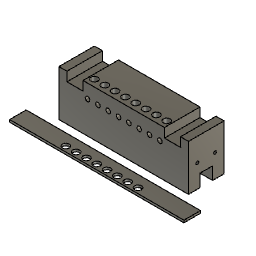
Simple_block_with_threaded_holes (Autodesk Fusion 360 design; units mm, degrees)
Autodesk Fusion 360 part; units mm, degrees
sketch "Sketch1" plane through (0, 0, 0) normal (0, 0, 1) x (1, 0, 0)
  line L0 (0, 0) -> (9, 0) construction
  line L1 (9, 0) -> (18, 0) construction
  line L2 (18, 0) -> (27, 0) construction
  line L3 (27, 0) -> (36, 0) construction
  line L4 (36, 0) -> (45, 0) construction
  line L5 (45, 0) -> (54, 0) construction
  line L6 (54, 0) -> (63, 0) construction
  line L7 (0, 0) -> (-25, 0) construction
  line L8 (63, 0) -> (88, 0) construction
  line L9 (-25, 0) -> (-25, -6) construction
  line L10 (88, 0) -> (88, -6) construction
  line L11 (88, -6) -> (-25, -6) construction
  line L12 (-25, 0) -> (-25, 25) construction
  line L13 (88, 0) -> (88, 25) construction
  line L14 (88, 25) -> (-25, 25) construction
  line L15 (88, -6) -> (-25, -6)
  line L16 (-25, -6) -> (-25, 25)
  line L17 (-25, 25) -> (88, 25)
  line L18 (88, 25) -> (88, -6)
  dimension "d1" = 9
  dimension "d2" = 9
  dimension "d3" = 9
  dimension "d4" = 9
  dimension "d5" = 9
  dimension "d6" = 9
  dimension "d7" = 9
  dimension "d8" = 25
  dimension "d9" = 25
  dimension "d10" = 6
  dimension "d11" = 6
  dimension "d12" = 25
  dimension "d13" = 25
  constraint coincident L0.start L7.start
  constraint horizontal L0
  constraint parallel L0 L1
  constraint parallel L1 L2
  constraint parallel L2 L3
  constraint parallel L3 L4
  constraint parallel L3 L5
  constraint parallel L3 L6
  constraint parallel L0 L7
  constraint parallel L6 L8
  constraint perpendicular L7 L9
  constraint perpendicular L8 L10
  constraint perpendicular L7 L12
  constraint perpendicular L8 L13
  measures "d1" distance of L0.start L0.end
  measures "d2" distance of L0.end L1.end
  measures "d3" distance of L1.end L2.end
  measures "d4" distance of L2.end L3.end
  measures "d5" distance of L3.end L4.end
  measures "d6" distance of L4.end L5.end
  measures "d7" distance of L5.end L6.end
  measures "d8" distance of L0.start L7.end
  measures "d9" distance of L6.end L8.end
  measures "d10" distance of L7.end L9.end
  measures "d11" distance of L8.end L10.end
  measures "d12" distance of L7.end L12.end
  measures "d13" distance of L8.end L13.end
  measures "d45" distance of L7.end
  measures "d53" diameter of L7.end
  measures "d91" distance of L7.end
extrude "Extrude1" add sketch "Sketch1" along normal blind 40 makes body 1
sketch "Sketch2" plane through (0, 0, 40) normal (0, 0, 1) x (-1, 0, 0)
  line L0 (-88, -25) -> (25, -25)
  line L1 (25, -25) -> (25, 6)
  line L2 (25, 6) -> (-88, 6)
  line L3 (-88, 6) -> (-88, -25)
  line L4 (25, 6) -> (25, 0) construction
  line L5 (25, 0) -> (0, 0) construction
  line L6 (0, 0) -> (-9, 0) construction
  line L7 (-9, 0) -> (-18, 0) construction
  line L8 (-18, 0) -> (-27, 0) construction
  line L9 (-27, 0) -> (-36, 0) construction
  line L10 (-36, 0) -> (-45, 0) construction
  line L11 (-45, 0) -> (-54, 0) construction
  line L12 (-54, 0) -> (-63, 0) construction
  line L13 (-63, 0) -> (-88, 0) construction
  circle A0 centre (0, 0) radius 3
  circle A1 centre (-9, 0) radius 3
  circle A2 centre (-18, 0) radius 3
  circle A3 centre (-27, 0) radius 3
  circle A4 centre (-36, 0) radius 3
  circle A5 centre (-45, 0) radius 3
  circle A6 centre (-54, 0) radius 3
  circle A7 centre (-63, 0) radius 3
  line L14 (0, 0) -> (4, 0) construction
  line L15 (0, 0) -> (18, 0) construction
  line L16 (-63, 0) -> (-81, 0) construction
  line L17 (-63, 0) -> (-67, 0) construction
  line L18 (-67, 0) -> (-67, 6) construction
  line L19 (-81, 0) -> (-81, 6) construction
  line L20 (-67, 6) -> (-67, -25)
  line L21 (-81, 6) -> (-81, -25)
  line L22 (18, 0) -> (18, 6) construction
  line L23 (4, 0) -> (4, 6) construction
  line L24 (18, 6) -> (18, -25)
  line L25 (4, 6) -> (4, -25)
  dimension "d16" = 6
  dimension "d17" = 25
  dimension "d18" = 9
  dimension "d19" = 9
  dimension "d20" = 9
  dimension "d21" = 9
  dimension "d22" = 9
  dimension "d23" = 9
  dimension "d24" = 9
  dimension "d25" = 6
  dimension "d26" = 6
  dimension "d27" = 6
  dimension "d28" = 6
  dimension "d29" = 6
  dimension "d30" = 6
  dimension "d31" = 6
  dimension "d32" = 6
  dimension "d56" = 4
  dimension "d57" = 18
  dimension "d58" = 18
  dimension "d59" = 4
  constraint coincident L1.end L2.start
  constraint perpendicular L2 L4
  constraint perpendicular L4 L5
  constraint perpendicular L4 L6
  constraint perpendicular L4 L7
  constraint parallel L7 L8
  constraint parallel L8 L9
  constraint parallel L9 L10
  constraint parallel L10 L11
  constraint parallel L11 L12
  constraint coincident L3 L13.end
  constraint perpendicular L3 L13
  constraint coincident L5.end L6.start
  constraint coincident L6.end L7.start
  constraint coincident L7.end L8.start
  constraint coincident L8.end L9.start
  constraint coincident L9.end L10.start
  constraint coincident L10.end L11.start
  constraint coincident L11.end L12.start
  constraint coincident L12.end L13.start
  constraint parallel L5 L14
  constraint parallel L5 L15
  constraint parallel L13 L16
  constraint parallel L13 L17
  constraint coincident L2 L18.end
  constraint perpendicular L2 L18
  constraint coincident L2 L19.end
  constraint perpendicular L2 L19
  constraint coincident L0 L20.end
  constraint perpendicular L0 L20
  constraint coincident L0 L21.end
  constraint perpendicular L0 L21
  constraint coincident L2 L22.end
  constraint perpendicular L2 L22
  constraint coincident L2 L23.end
  constraint perpendicular L2 L23
  constraint coincident L0 L24.end
  constraint perpendicular L0 L24
  constraint coincident L0 L25.end
  constraint perpendicular L0 L25
  measures "d16" distance of L1.end L4.end
  measures "d17" distance of L4.end L5.end
  measures "d18" distance of L5.end L6.end
  measures "d19" distance of L6.end L7.end
  measures "d20" distance of L7.end L8.end
  measures "d21" distance of L8.end L9.end
  measures "d22" distance of L9.end L10.end
  measures "d23" distance of L10.end L11.end
  measures "d24" distance of L11.end L12.end
  measures "d25" diameter of A0
  measures "d26" diameter of A1
  measures "d27" diameter of A2
  measures "d28" diameter of A3
  measures "d29" diameter of A4
  measures "d30" diameter of A5
  measures "d31" diameter of A6
  measures "d32" diameter of A7
  measures "d56" distance of L5.end L14.end
  measures "d57" distance of L5.end L15.end
  measures "d58" distance of L12.end L16.end
  measures "d59" distance of L12.end L17.end
sketch "Sketch3" plane through (0, -6, 0) normal (0, -1, 0) x (1, 0, 0)
  line L0 (-25, 0) -> (88, 0)
  line L1 (88, 0) -> (88, 40)
  line L2 (88, 40) -> (-25, 40)
  line L3 (-25, 40) -> (-25, 0)
  line L4 (-25, 40) -> (0, 40) construction
  line L5 (0, 40) -> (9, 40) construction
  line L6 (9, 40) -> (18, 40) construction
  line L7 (18, 40) -> (27, 40) construction
  line L8 (27, 40) -> (36, 40) construction
  line L9 (36, 40) -> (45, 40) construction
  line L10 (45, 40) -> (54, 40) construction
  line L11 (54, 40) -> (63, 40) construction
  line L12 (63, 40) -> (88, 40) construction
  line L13 (0, 40) -> (0, 28) construction
  line L14 (63, 40) -> (63, 28) construction
  line L15 (63, 28) -> (0, 28) construction
  line L16 (9, 40) -> (9, 28) construction
  line L17 (18, 40) -> (18, 28) construction
  line L18 (27, 40) -> (27, 28) construction
  line L19 (36, 40) -> (36, 28) construction
  line L20 (45, 40) -> (45, 28) construction
  line L21 (54, 40) -> (54, 28) construction
  circle A0 centre (0, 28) radius 2
  circle A1 centre (9, 28) radius 2
  circle A2 centre (18, 28) radius 2
  circle A3 centre (27, 28) radius 2
  circle A4 centre (36, 28) radius 2
  circle A5 centre (45, 28) radius 2
  circle A6 centre (54, 28) radius 2
  circle A7 centre (63, 28) radius 2
  dimension "d33" = 25
  dimension "d34" = 9
  dimension "d35" = 9
  dimension "d36" = 9
  dimension "d37" = 9
  dimension "d38" = 9
  dimension "d39" = 9
  dimension "d40" = 9
  dimension "d44" = 12
  dimension "d45" = 12
  dimension "d46" = 4
  dimension "d47" = 4
  dimension "d48" = 4
  dimension "d49" = 4
  dimension "d50" = 4
  dimension "d51" = 4
  dimension "d52" = 4
  dimension "d53" = 4
  constraint coincident L2.end L3.start
  constraint perpendicular L3 L4
  constraint perpendicular L3 L5
  constraint coincident L2 L6.end
  constraint parallel L2 L7
  constraint parallel L2 L8
  constraint parallel L2 L9
  constraint parallel L2 L10
  constraint parallel L2 L11
  constraint coincident L1.end L2.start
  constraint perpendicular L4 L13
  constraint perpendicular L11 L14
  constraint coincident L15 L16.end
  constraint perpendicular L15 L16
  constraint coincident L15 L17.end
  constraint perpendicular L15 L17
  constraint coincident L15 L18.end
  constraint perpendicular L15 L18
  constraint coincident L15 L19.end
  constraint perpendicular L15 L19
  constraint coincident L15 L20.end
  constraint perpendicular L15 L20
  constraint coincident L15 L21.end
  constraint perpendicular L15 L21
  constraint coincident L13.end L15.end
  constraint coincident L16.end A1.centre
  constraint coincident L17.end A2.centre
  constraint coincident L18.end A3.centre
  constraint coincident L19.end A4.centre
  constraint coincident L20.end A5.centre
  constraint coincident L21.end A6.centre
  constraint coincident L14.end L15.start
  measures "d33" distance of L2.end L4.end
  measures "d34" distance of L4.end L5.end
  measures "d35" distance of L5.end L6.end
  measures "d36" distance of L6.end L7.end
  measures "d37" distance of L7.end L8.end
  measures "d38" distance of L8.end L9.end
  measures "d39" distance of L9.end L10.end
  measures "d40" distance of L10.end L11.end
  measures "d44" distance of L4.end L13.end
  measures "d45" distance of L11.end L14.end
  measures "d46" diameter of A0
  measures "d47" diameter of A1
  measures "d48" diameter of A2
  measures "d49" diameter of A3
  measures "d50" diameter of A4
  measures "d51" diameter of A5
  measures "d52" diameter of A6
  measures "d53" diameter of A7
extrude "Extrude2" cut sketch "Sketch2" against normal blind 14 contours A0 | A1 | A2 | A3 | A4 | A5 | A6 | A7 bodies 1
extrude "Extrude3" cut sketch "Sketch3" against normal blind 6 contours A0 | A1 | A2 | A3 | A4 | A5 | A6 | A7 bodies 1
extrude "Extrude4" cut sketch "Sketch2" against normal blind 8 contours L0 L2 L20 L21 | L0 L2 L24 L25 bodies 1
sketch "Sketch4" plane through (88, 0, 0) normal (1, 0, 0) x (0, 1, 0)
  line L0 (-6, 0) -> (25, 0)
  line L1 (25, 0) -> (25, 40)
  line L2 (25, 40) -> (-6, 40)
  line L3 (-6, 40) -> (-6, 0)
  line L4 (9.5, 0) -> (9.5, 11) construction
  line L5 (9.5, 11) -> (15, 11) construction
  line L6 (15, 11) -> (9.5, 11) construction
  line L7 (9.5, 11) -> (4, 11) construction
  line L8 (4, 11) -> (4, 0)
  line L9 (15, 11) -> (15, 0)
  line L10 (15, 11) -> (4, 11)
  dimension "d62" = 11
  dimension "d63" = 5.5
  dimension "d64" = 5.5
  constraint midpoint L0 L4.start
  constraint perpendicular L0 L4
  constraint perpendicular L4 L5
  constraint perpendicular L4 L7
  constraint coincident L0 L8.end
  constraint perpendicular L0 L8
  constraint coincident L0 L9.end
  constraint perpendicular L0 L9
  measures "d62" distance of L4.start L4.end
  measures "d63" distance of L4.end L5.end
  measures "d64" distance of L4.end L7.end
extrude "Extrude5" cut sketch "Sketch4" against normal blind 113 contours L0 L8 L9 L10 bodies 1
sketch "Sketch5" plane through (88, 0, 0) normal (1, 0, 0) x (0, 1, 0)
  line L0 (15, 11) -> (15, 0)
  line L1 (15, 0) -> (25, 0)
  line L2 (25, 0) -> (25, 40)
  line L3 (25, 40) -> (-6, 40)
  line L4 (-6, 40) -> (-6, 0)
  line L5 (-6, 0) -> (4, 0)
  line L6 (4, 0) -> (4, 11)
  line L7 (4, 11) -> (15, 11)
  line L8 (-6, 40) -> (-6, 20) construction
  line L9 (-6, 20) -> (25, 20) construction
  line L10 (9.5, 20) -> (-6, 20) construction
  line L11 (9.5, 20) -> (25, 20) construction
  circle A0 centre (17.25, 20) radius 1.25
  circle A1 centre (1.75, 20) radius 1.25
  dimension "d67" = 20
  dimension "d68" = 2.5
  dimension "d69" = 2.5
  constraint coincident L3.end L4.start
  constraint midpoint L4 L8.end
  constraint midpoint L2 L9.end
  constraint midpoint L9 L10.start
  constraint midpoint L11 A0.centre
  constraint midpoint L10 A1.centre
  measures "d67" distance of L3.end L8.end
  measures "d68" diameter of A0
  measures "d69" diameter of A1
extrude "Extrude6" cut sketch "Sketch5" against normal blind 15 contours A0 | A1 bodies 1
sketch "Sketch6" plane through (-25, 0, 0) normal (-1, 0, 0) x (0, -1, 0)
  line L0 (-15, 0) -> (-15, 11)
  line L1 (-15, 11) -> (-4, 11)
  line L2 (-4, 11) -> (-4, 0)
  line L3 (-4, 0) -> (6, 0)
  line L4 (6, 0) -> (6, 40)
  line L5 (6, 40) -> (-25, 40)
  line L6 (-25, 40) -> (-25, 0)
  line L7 (-25, 0) -> (-15, 0)
  line L8 (-25, 40) -> (-25, 20) construction
  line L9 (-25, 20) -> (6, 20) construction
  line L10 (-9.5, 20) -> (6, 20) construction
  line L11 (-9.5, 20) -> (-25, 20) construction
  circle A0 centre (-17.25, 20) radius 1.25
  circle A1 centre (-1.75, 20) radius 1.25
  dimension "d72" = 20
  dimension "d73" = 2.5
  dimension "d74" = 2.5
  constraint coincident L5.end L6.start
  constraint perpendicular L5 L8
  constraint midpoint L4 L9.end
  constraint midpoint L9 L10.start
  constraint midpoint L11 A0.centre
  constraint midpoint L10 A1.centre
  measures "d72" distance of L5.end L8.end
  measures "d73" diameter of A0
  measures "d74" diameter of A1
extrude "Extrude7" cut sketch "Sketch6" against normal blind 15 contours A0 | A1 bodies 1
sketch "Sketch1 (2)" plane through (0, 0, 0) normal (0, 0, 1) x (1, 0, 0) in component "Lid"
  line L0 (0, -25) -> (9, -25) construction
  line L1 (9, -25) -> (18, -25) construction
  line L2 (18, -25) -> (27, -25) construction
  line L3 (27, -25) -> (36, -25) construction
  line L4 (36, -25) -> (45, -25) construction
  line L5 (45, -25) -> (54, -25) construction
  line L6 (54, -25) -> (63, -25) construction
  line L7 (63, -25) -> (63, -29.5) construction
  line L8 (0, -25) -> (0, -29.5) construction
  line L9 (0, -25) -> (0, -15) construction
  line L10 (63, -25) -> (63, -15) construction
  line L11 (0, -25) -> (-4.5, -25) construction
  line L12 (-4.5, -25) -> (-44.5, -25) construction
  line L13 (63, -25) -> (67.5, -25) construction
  line L14 (67.5, -25) -> (107.5, -25) construction
  line L15 (107.5, -25) -> (107.5, -29.5) construction
  line L16 (-44.5, -25) -> (-44.5, -29.5) construction
  line L17 (-44.5, -25) -> (-44.5, -15) construction
  line L18 (107.5, -25) -> (107.5, -15) construction
  line L19 (107.5, -15) -> (107.5, -29.5)
  line L20 (-44.5, -29.5) -> (-44.5, -15)
  line L21 (-44.5, -29.5) -> (107.5, -29.5)
  line L22 (107.5, -15) -> (-44.5, -15)
  circle A0 centre (0, -25) radius 3
  circle A1 centre (9, -25) radius 3
  circle A2 centre (18, -25) radius 3
  circle A3 centre (27, -25) radius 3
  circle A4 centre (36, -25) radius 3
  circle A5 centre (45, -25) radius 3
  circle A6 centre (54, -25) radius 3
  circle A7 centre (63, -25) radius 3
  dimension "d77" = 9
  dimension "d78" = 9
  dimension "d79" = 9
  dimension "d80" = 9
  dimension "d81" = 9
  dimension "d82" = 9
  dimension "d83" = 9
  dimension "d84" = 4.5
  dimension "d85" = 4.5
  dimension "d86" = 10
  dimension "d87" = 10
  dimension "d88" = 4.5
  dimension "d89" = 40
  dimension "d90" = 4.5
  dimension "d91" = 40
  dimension "d92" = 4.5
  dimension "d93" = 4.5
  dimension "d94" = 10
  dimension "d95" = 10
  dimension "d96" = 6
  dimension "d97" = 6
  dimension "d98" = 6
  dimension "d99" = 6
  dimension "d100" = 6
  dimension "d101" = 6
  dimension "d102" = 6
  dimension "d103" = 6
  constraint horizontal L0
  constraint parallel L0 L1
  constraint parallel L1 L2
  constraint parallel L2 L3
  constraint parallel L3 L4
  constraint parallel L4 L5
  constraint parallel L5 L6
  constraint perpendicular L6 L7
  constraint perpendicular L0 L8
  constraint perpendicular L0 L9
  constraint perpendicular L6 L10
  constraint perpendicular L9 L11
  constraint perpendicular L9 L12
  constraint perpendicular L7 L13
  constraint perpendicular L7 L14
  constraint perpendicular L14 L15
  constraint perpendicular L12 L16
  constraint perpendicular L12 L17
  constraint perpendicular L14 L18
  constraint coincident L0.start L8.start
  constraint coincident L0.end L1.start
  constraint coincident L1.end L2.start
  constraint coincident L2.end L3.start
  constraint coincident L3.end L4.start
  constraint coincident L4.end L5.start
  constraint coincident L5.end L6.start
  constraint coincident L6.end L7.start
  measures "d77" distance of L0.start L0.end
  measures "d78" distance of L0.end L1.end
  measures "d79" distance of L1.end L2.end
  measures "d80" distance of L2.end L3.end
  measures "d81" distance of L3.end L4.end
  measures "d82" distance of L4.end L5.end
  measures "d83" distance of L5.end L6.end
  measures "d84" distance of L6.end L7.end
  measures "d85" distance of L0.start L8.end
  measures "d86" distance of L0.start L9.end
  measures "d87" distance of L6.end L10.end
  measures "d88" distance of L0.start L11.end
  measures "d89" distance of L11.end L12.end
  measures "d90" distance of L6.end L13.end
  measures "d91" distance of L13.end L14.end
  measures "d92" distance of L14.end L15.end
  measures "d93" distance of L12.end L16.end
  measures "d94" distance of L12.end L17.end
  measures "d95" distance of L14.end L18.end
  measures "d96" diameter of A0
  measures "d97" diameter of A1
  measures "d98" diameter of A2
  measures "d99" diameter of A3
  measures "d100" diameter of A4
  measures "d101" diameter of A5
  measures "d102" diameter of A6
  measures "d103" diameter of A7
extrude "Extrude1'" add sketch "Sketch1 (2)" along normal blind 2 separate body makes body 2 in component "Lid"
sketch "Sketch7" plane through (0, -6, 0) normal (0, -1, 0) x (1, 0, 0)
  line L0 (81, 40) -> (81, 32)
  line L1 (81, 32) -> (67, 32)
  line L2 (67, 32) -> (67, 40)
  line L3 (67, 40) -> (-4, 40)
  line L4 (-4, 40) -> (-4, 32)
  line L5 (-4, 32) -> (-18, 32)
  line L6 (-18, 32) -> (-18, 40)
  line L7 (-18, 40) -> (-25, 40)
  line L8 (-25, 40) -> (-25, 0)
  line L9 (-25, 0) -> (88, 0)
  line L10 (88, 0) -> (88, 40)
  line L11 (88, 40) -> (81, 40)
  circle A0 centre (63, 28) radius 2
  circle A1 centre (27, 28) radius 2
  circle A2 centre (0, 28) radius 2
  circle A3 centre (36, 28) radius 2
  circle A4 centre (54, 28) radius 2
  circle A5 centre (18, 28) radius 2
  circle A6 centre (9, 28) radius 2
  circle A7 centre (45, 28) radius 2
  dimension "d106" = 71
  dimension "d107" = 113
  dimension "d108" = 40
  dimension "d109" = 14
  dimension "d110" = 7
  dimension "d111" = 8
  dimension "d122" = 28
  dimension "d123" = 12
  dimension "d124" = 9
  dimension "d125" = 25
  dimension "d126" = 4
  dimension "d127" = 9
  dimension "d128" = 9
  measures "d106" distance of L2.end L3.end
  measures "d107" distance of L8.end L9.end
  measures "d108" distance of L9.end L10.end
  measures "d109" distance of L0.end L1.end
  measures "d110" distance of L0.start L10.end
  measures "d111" distance of L1 L3
  measures "d122" distance of L9 A0.centre
  measures "d123" distance of L3 A0.centre
  measures "d124" distance of A1.centre A3.centre
  measures "d125" distance of L8 A2.centre
  measures "d126" diameter of A6
  measures "d127" distance of A3.centre A7.centre
  measures "d128" distance of A4.centre A7.centre
sketch "Sketch8" plane through (88, 0, 0) normal (1, 0, 0) x (0, 1, 0)
  circle A0 centre (1.75, 20) radius 1.25
  circle A1 centre (17.25, 20) radius 1.25
  line L0 (15, 11) -> (15, 0)
  line L1 (15, 0) -> (25, 0)
  line L2 (25, 0) -> (25, 40)
  line L3 (25, 40) -> (-6, 40)
  line L4 (-6, 40) -> (-6, 0)
  line L5 (-6, 0) -> (4, 0)
  line L6 (4, 0) -> (4, 11)
  line L7 (4, 11) -> (15, 11)
  line L8 (-6, 0) -> (-6, 40)
  dimension "d112" = 31
  dimension "d113" = 11
  dimension "d114" = 10
  dimension "d115" = 40
  dimension "d116" = 7.75
  dimension "d117" = 20
  dimension "d118" = 20
  dimension "d119" = 15.5
  dimension "d120" = 7.75
  dimension "d121" = 11
  measures "d112" distance of L2.end L3.end
  measures "d113" distance of L0.start L6.end
  measures "d114" distance of L0.end L1.end
  measures "d115" distance of L1.end L2.end
  measures "d116" distance of A1.centre L2
  measures "d117" distance of A1.centre L3
  measures "d118" distance of A1.centre L1
  measures "d119" distance of A0.centre A1.centre
  measures "d120" distance of A0.centre L8
  measures "d121" distance of L5 L7
sketch "Sketch9" plane through (0, 0, 40) normal (0, 0, 1) x (-1, 0, 0)
  line L0 (-67, 6) -> (-67, -25)
  line L1 (-67, -25) -> (4, -25)
  line L2 (4, -25) -> (4, 6)
  line L3 (4, 6) -> (-67, 6)
  circle A0 centre (-9, 0) radius 3
  circle A1 centre (-54, 0) radius 3
  circle A2 centre (-45, 0) radius 3
  circle A3 centre (-18, 0) radius 3
  circle A4 centre (0, 0) radius 3
  circle A5 centre (-63, 0) radius 3
  circle A6 centre (-36, 0) radius 3
  circle A7 centre (-27, 0) radius 3
  line L4 (-88, -25) -> (-81, -25)
  line L5 (-88, -25) -> (-88, 6)
  line L6 (-67, -25) -> (-81, -25)
  line L7 (25, -25) -> (25, 6)
  dimension "d129" = 7
  dimension "d130" = 71
  dimension "d131" = 31
  dimension "d132" = 14
  dimension "d133" = 4
  dimension "d134" = 9
  dimension "d135" = 6
  dimension "d136" = 25
  dimension "d137" = 9
  dimension "d138" = 6
  dimension "d139" = 113
  measures "d129" distance of L4.start L4.end
  measures "d130" distance of L0.end L1.end
  measures "d131" distance of L4.start L5.end
  measures "d132" distance of L0.end L4.end
  measures "d133" distance of A4.centre L2
  measures "d134" distance of A4.centre A0.centre
  measures "d135" distance of A4.centre L3
  measures "d136" distance of A4.centre L1
  measures "d137" distance of A0.centre A3.centre
  measures "d138" diameter of A0
  measures "d139" distance of L5 L7
sketch "Sketch10" plane through (0, 0, 2) normal (0, 0, 1) x (-1, 0, 0)
  circle A0 centre (-18, 25) radius 3
  circle A1 centre (-54, 25) radius 3
  circle A2 centre (-36, 25) radius 3
  circle A3 centre (-9, 25) radius 3
  circle A4 centre (-45, 25) radius 3
  circle A5 centre (-63, 25) radius 3
  circle A6 centre (-27, 25) radius 3
  circle A7 centre (0, 25) radius 3
  line L0 (44.5, 29.5) -> (-107.5, 29.5)
  line L1 (-107.5, 29.5) -> (-107.5, 15)
  line L2 (-107.5, 15) -> (44.5, 15)
  line L3 (44.5, 15) -> (44.5, 29.5)
  dimension "d140" = 152
  dimension "d141" = 14.5
  dimension "d142" = 44.5
  dimension "d143" = 4.5
  dimension "d144" = 10
  dimension "d145" = 9
  dimension "d146" = 9
  measures "d140" distance of L1.end L2.end
  measures "d141" distance of L0.end L1.end
  measures "d142" distance of A5.centre L1
  measures "d143" distance of A7.centre L0
  measures "d144" distance of A5.centre L2
  measures "d145" distance of A3.centre A7.centre
  measures "d146" distance of A0.centre A3.centre
sketch "Sketch11" plane through (0, -29.5, 0) normal (0, -1, 0) x (1, 0, 0)
  line L0 (-44.5, 0) -> (107.5, 0)
  line L1 (107.5, 0) -> (107.5, 2)
  line L2 (107.5, 2) -> (-44.5, 2)
  line L3 (-44.5, 2) -> (-44.5, 0)
  dimension "d147" = 152
  dimension "d148" = 2
  measures "d147" distance of L0.start L0.end
  measures "d148" distance of L0.end L1.end
sketch "Sketch12" plane through (0, 0, 0) normal (0, 0, -1) x (1, 0, 0)
  line L0 (-25, -4) -> (88, -4)
  line L1 (88, -4) -> (88, 6)
  line L2 (88, 6) -> (-25, 6)
  line L3 (-25, 6) -> (-25, -4)
  line L4 (-25, 1) -> (88, 1) construction
  line L5 (31.5, 6) -> (88, 6) construction
  line L6 (31.5, 6) -> (-25, 6) construction
  line L7 (3.25, 6) -> (3.25, -4) construction
  line L8 (59.75, 6) -> (59.75, -4) construction
  circle A0 centre (3.25, 1) radius 1.25
  circle A1 centre (59.75, 1) radius 1.25
  dimension "d149" = 2.5
  dimension "d150" = 2.5
  constraint midpoint L3 L4.start
  constraint midpoint L1 L4.end
  constraint midpoint L2 L5.start
  constraint coincident L1.end L2.start
  constraint coincident L2.end L3.start
  constraint midpoint L6 L7.start
  constraint coincident L0 L7.end
  constraint perpendicular L0 L7
  constraint midpoint L5 L8.start
  constraint coincident L0 L8.end
  constraint perpendicular L0 L8
  constraint midpoint L7 A0.centre
  constraint midpoint L8 A1.centre
  measures "d149" diameter of A0
  measures "d150" diameter of A1
sketch "Sketch13" plane through (0, 0, 0) normal (0, 0, -1) x (1, 0, 0)
  line L0 (88, -15) -> (-25, -15)
  line L1 (-25, -15) -> (-25, -25)
  line L2 (-25, -25) -> (88, -25)
  line L3 (88, -25) -> (88, -15)
  line L4 (-25, -20) -> (88, -20) construction
  line L5 (31.5, -25) -> (-25, -25) construction
  line L6 (31.5, -25) -> (88, -25) construction
  line L7 (3.25, -25) -> (3.25, -15) construction
  line L8 (59.75, -25) -> (59.75, -15) construction
  circle A0 centre (3.25, -20) radius 1.25
  circle A1 centre (59.75, -20) radius 1.25
  dimension "d151" = 2.5
  dimension "d152" = 2.5
  constraint midpoint L1 L4.start
  constraint midpoint L3 L4.end
  constraint midpoint L2 L5.start
  constraint coincident L1.end L2.start
  constraint coincident L2.end L3.start
  constraint midpoint L5 L7.start
  constraint coincident L0 L7.end
  constraint perpendicular L0 L7
  constraint midpoint L6 L8.start
  constraint coincident L0 L8.end
  constraint perpendicular L0 L8
  constraint midpoint L7 A0.centre
  constraint midpoint L8 A1.centre
  measures "d151" diameter of A0
  measures "d152" diameter of A1
sketch "Sketch14" plane through (0, 0, 0) normal (0, 0, -1) x (1, 0, 0)
  line L0 (88, -15) -> (-25, -15)
  line L1 (-25, -15) -> (-25, -25)
  line L2 (-25, -25) -> (88, -25)
  line L3 (88, -25) -> (88, -15)
extrude "Extrude8" cut sketch "Sketch13" sketch "Sketch12" against normal blind 15 contours A0 | A1 of sketch 2 contours A0 | A1 bodies 1
sketch "Sketch15" plane through (0, 25, 0) normal (0, 1, 0) x (-1, 0, 0)
  line L0 (-81, 32) -> (-81, 40)
  line L1 (-81, 40) -> (-88, 40)
  line L2 (-88, 40) -> (-88, 0)
  line L3 (-88, 0) -> (25, 0)
  line L4 (25, 0) -> (25, 40)
  line L5 (25, 40) -> (18, 40)
  line L6 (18, 40) -> (18, 32)
  line L7 (18, 32) -> (4, 32)
  line L8 (4, 32) -> (4, 40)
  line L9 (4, 40) -> (-67, 40)
  line L10 (-67, 40) -> (-67, 32)
  line L11 (-67, 32) -> (-81, 32)
sketch "Sketch16" plane through (0, 0, 0) normal (0, 0, -1) x (1, 0, 0)
  circle A0 centre (59.75, 1) radius 1.25
  circle A1 centre (3.25, 1) radius 1.25
  line L0 (-25, -4) -> (88, -4)
  line L1 (88, -4) -> (88, 6)
  line L2 (88, 6) -> (-25, 6)
  line L3 (-25, 6) -> (-25, -4)
  line L4 (88, 6) -> (88, -4)
  dimension "d155" = 28.25
  dimension "d156" = 5
  dimension "d157" = 5
  dimension "d158" = 28.25
  measures "d155" distance of A1.centre L3
  measures "d156" distance of A1.centre L2
  measures "d157" distance of A0.centre L2
  measures "d158" distance of A0.centre L4
sketch "Sketch17" plane through (0, 0, 0) normal (0, 0, -1) x (1, 0, 0)
component "Lid" placed x (1, 0, 0) y (0, 1, 0) z (0, 0, 1) at (0, 0, 0)
